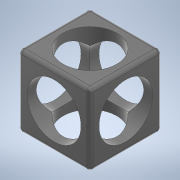
# Autodesk Inventor part: КубСоединительный2020
Saved by Autodesk Inventor 2020 (Build 240168000, 168)
## iProperties
Created: 2019-11-02
Part Number: КубСоединительный2020
Material: Типовые
Document SubType Name: Modeling
Designer: Михаил
Density: 1 g/cm^3
Appearance: По умолчанию
Author: Михаил
Autodesk Inventor part; units mm, degrees
ref_plane "YZ Plane" through (0, 0, 0) normal (1, 0, 0) x (0, 1, 0)
ref_plane "XZ Plane" through (0, 0, 0) normal (0, 1, 0) x (-1, 0, 0)
ref_plane "XY Plane" through (0, 0, 0) normal (0, 0, 1) x (1, 0, 0)
sketch "Эскиз1" plane through (0, 0, 0) normal (0, 1, 0) x (-1, 0, 0)
  line L0 (0, 0) -> (20, 0)
  line L1 (20, 0) -> (20, -20)
  line L2 (20, -20) -> (0, -20)
  line L3 (0, -20) -> (0, 0)
  dimension "d0" = 20
  dimension "d1" = 20
  constraints: 8 end point, 2 parallel, 1 horizontal, 1 perpendicular
  measures "d0" distance of L2.end L1.end
  measures "d1" distance of L2.end L0.start
extrude "Выдавливание1" add sketch "Эскиз1" along normal blind 20
sketch "Эскиз2" plane through (0, 20, 0) normal (0, 1, 0) x (1, 0, 0)
  circle A0 centre (-10, 10) radius 7.5
  line L0 (0, 0) -> (0, 20) projected
  dimension "d4" = 15
  dimension "d5" = 10
  dimension "d6" = 10
  constraints: 1 centre point
  measures "d4" diameter of A0
  measures "d5" horizontal distance of L0.start A0.centre
  measures "d6" distance from line of L0 A0.centre
sketch "Эскиз3" plane through (0, 0, -20) normal (0, 0, -1) x (-1, 0, 0)
  circle A0 centre (10, 10) radius 7.5
  line L0 (0, 0) -> (0, 20) projected
  line L1 (0, 0) -> (20, 0) projected
  dimension "d7" = 15
  dimension "d8" = 10
  dimension "d9" = 10
  constraints: 1 centre point
  measures "d7" diameter of A0
  measures "d8" distance from line of L0 A0.centre
  measures "d9" distance from line of L1 A0.centre
sketch "Эскиз4" plane through (0, 0, 0) normal (1, 0, 0) x (0, 0, -1)
  circle A0 centre (10, 10) radius 7.5
  line L0 (20, 0) -> (20, 20) projected
  line L1 (0, 20) -> (20, 20) projected
  point P0 (0, 0)
  dimension "d10" = 15
  dimension "d11" = 10
  dimension "d12" = 10
  constraints: 1 centre point
  measures "d10" diameter of A0
  measures "d11" distance from line of L0 A0.centre
  measures "d12" distance from line of L1 A0.centre
extrude "Выдавливание2" cut sketch "Эскиз2" against normal blind 20
extrude "Выдавливание3" cut sketch "Эскиз4" against normal blind 20
extrude "Выдавливание4" cut sketch "Эскиз3" against normal blind 20
fillet "Сопряжение1" radius 1 12 edges at (0, 0, -10) (-10, 0, -20) (0, 10, -20) (0, 20, -10) (-10, 20, -20) (-20, 20, -10) (-20, 0, -10) (-10, 0, 0) (-10, 20, 0) (0, 10, 0) (-20, 10, 0) (-20, 10, -20)
